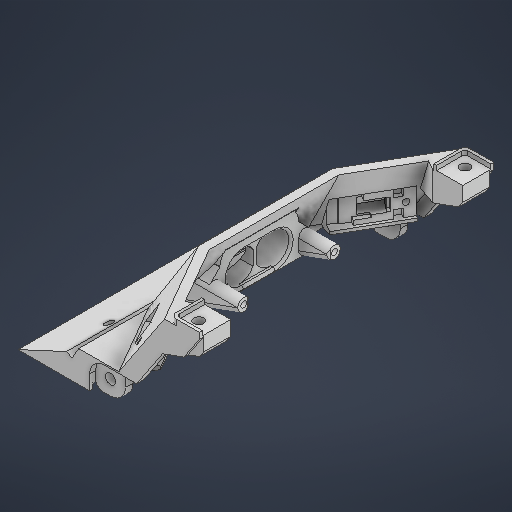
# Autodesk Inventor part: body-front
Saved by Autodesk Inventor 2025 (Build 290162000, 162)
## iProperties
Created: 2025-03-18
Part Number: body-front
Material: Všeobecné
Document SubType Name: Modeling
Designer: Simak
Density: 1 g/cm^3
Appearance: Výchozí
Author: Simak
Autodesk Inventor part; units mm, degrees
ref_plane "XZ Plane" through (0, 0, 0) normal (0, 1, 0) x (-1, 0, 0)
sketch "Náčrt1" plane through (0, 0, 0) normal (0, 0, 1) x (1, 0, 0)
  line L0 (29.0793, 0) -> (0, 0)
  line L1 (18.1093, 6.5703) -> (33.6572, 33.5)
  line L2 (33.6572, 33.5) -> (60.9683, 33.5)
  line L3 (60.9683, 33.5) -> (60.9683, 26.6) construction
  circle A0 centre (74.2183, 13.5) radius 16.5 construction
  line L4 (15.7407, 11.2018) -> (-8.2817, 0) construction
  line L5 (-8.2817, 0) -> (0, 0) construction
  line L6 (52.2183, 35.6) -> (89.7183, 35.6) construction
  line L7 (89.7183, 35.6) -> (89.7183, 34) construction
  line L8 (89.7183, 34) -> (52.2183, 34) construction
  line L9 (52.2183, 34) -> (52.2183, 35.6) construction
  line L10 (55.9683, 35.6) -> (55.9683, 34) construction
  circle A1 centre (74.2183, 15.5) radius 16.5
  circle A2 centre (74.2183, 11.5) radius 16.5
  line L11 (57.7183, 15.5) -> (57.7183, 11.5)
  line L12 (74.2183, 15.5) -> (74.2183, 13.5) construction
  line L13 (74.2183, 13.5) -> (74.2183, 11.5) construction
  line L14 (70.6632, 32.5) -> (65.9683, 29.7894)
  line L15 (70.6632, 33.5) -> (60.9683, 33.5)
  line L16 (70.6632, 33.5) -> (70.6632, 32.5)
  line L17 (62.0101, 26.6) -> (32.5602, 26.6)
  line L18 (10.0793, 4.2) -> (10.0793, 2.6) construction
  line L19 (20.5793, 4.2) -> (10.0793, 4.2) construction
  line L20 (11.4205, 8.6356) -> (13.8505, 3.4243) construction
  line L21 (13.8505, 3.4243) -> (12.7622, 0.4342) construction
  line L22 (12.7622, 0.4342) -> (19.5595, 3.6039) construction
  line L23 (19.5595, 3.6039) -> (16.5694, 4.6922) construction
  line L24 (16.5694, 4.6922) -> (14.1394, 9.9034) construction
  line L25 (14.1394, 9.9034) -> (11.4205, 8.6356) construction
  line L26 (10.0793, 2.6) -> (20.5793, 2.6) construction
  line L27 (20.5793, 2.6) -> (20.5793, 4.2) construction
  line L28 (20.5793, 4.2) -> (23.5793, 4.2) construction
  line L29 (23.5793, 4.2) -> (23.5793, 2.6) construction
  line L30 (23.5793, 2.6) -> (20.5793, 2.6) construction
  line L31 (19.5595, 3.6039) -> (21.24, 0) construction
  line L32 (0, 0) -> (16.3135, 7.6071)
  line L33 (16.3135, 7.6071) -> (18.1093, 6.5703)
  circle A3 centre (29.0793, 5) radius 5
  line L34 (22.9762, 10) -> (32.5602, 26.6)
  line L35 (22.9762, 10) -> (29.0793, 10)
  line L36 (15.7407, 11.2018) -> (17.2198, 8.0297) construction
  line L37 (17.2198, 8.0297) -> (16.3135, 7.6071) construction
  line L38 (22.9762, 10) -> (17.2027, 0)
  line L39 (34.0793, 5) -> (34.0793, 10.5)
  line L40 (34.0793, 10.5) -> (23.2649, 10.5)
  line L41 (32.5602, 26.6) -> (36.5439, 33.5)
  point P0 (90.7183, 13.5)
  dimension "d2" = 33
  dimension "d3" = 13.5
  dimension "d6" = 99
  dimension "d8" = 1.6
  dimension "d9" = 37.5
  dimension "d10" = 3.75
  dimension "d11" = 4
  dimension "d12" = 1
  dimension "d13" = 0.5
  dimension "d14" = 5
  dimension "d17" = 4
  dimension "d18" = 60
  dimension "d19" = 1
  dimension "d20" = 9
  dimension "d21" = 60
  dimension "d23" = 4.2
  dimension "d24" = 1.6
  dimension "d27" = 45
  dimension "d29" = 3
  dimension "d31" = 8
  dimension "d32" = 7.5
  dimension "d37" = 0.5
  dimension "d38" = 3
  dimension "d40" = 25
  dimension "d41" = 1
  dimension "d44" = 10.5
  dimension "d45" = 3.5
  dimension "d46" = 0.5
  dimension "d47" = 10
  dimension "d48" = 11.2018
  dimension "d49" = 0.5
  dimension "d50" = 2.5
  dimension "d58" = 19
  dimension "d59" = 1.5
  dimension "d65" = 2
  dimension "d80" = 18.361
  dimension "d86" = 10.5
  dimension "d336" = 45.139
  constraints: 85 end point, 15 perpendicular, 8 horizontal, 8 point on line, 6 point on circle, 5 tangent, 4 collinear, 4 parallel, 4 vertical, 3 equal length, 3 horizontal alignment, 2 centre point, 2 vertical alignment, 6 other
  measures "d3" distance from line of L0 L12.end
  measures "d6" horizontal distance of L4.end point (90.718, 13.5)
  measures "d8" distance of L6.end L7.end
  measures "d9" distance of L6.start L6.end
  measures "d10" distance between parallel lines of L9 L10
  measures "d12" distance from line of point (90.718, 13.5) L7
  measures "d13" distance between parallel lines of L8 L2
  measures "d14" distance between parallel lines of L10 L3
  measures "d17" distance of L13.end L12.start
  measures "d18" angle of L3 L14
  measures "d19" distance of L15.start L14.start
  measures "d20" distance between parallel lines of L6 L17
  measures "d21" angle of L0 L1
  measures "d23" distance between parallel lines of L0 L19
  measures "d24" distance of L18.start L18.end
  measures "d27" angle of L22 L23
  measures "d29" distance of L24.end L20.start
  measures "d31" distance from line of L24.end L22
  measures "d32" distance of L21.end L22.end
  measures "d37" distance from line of L31 L26.end
  measures "d38" distance of L19.start L28.end
  measures "d40" angle of L0 L32
  measures "d41" distance from line of L24 L32.end
  measures "d44" distance of L19.start L18.start
  measures "d45" distance between parallel lines of L32 L4
  measures "d46" distance between parallel lines of L4 L25
  measures "d47" diameter of A3
  measures "d48" distance from line of L0 L4.start
  measures "d49" distance edge to line of A3 L29
  measures "d50" distance between parallel lines of L1 L34
  measures "d58" distance from line of L0.end L36
  measures "d59" distance from line of L36.end L1
  measures "d65" distance between parallel lines of L36 L24
  measures "d80" horizontal distance of L4.end L18.end
  measures "d86" distance between parallel lines of L0 L40
  measures "d336" horizontal distance of A3.centre L12.end
extrude "Vysunutí1" add sketch "Náčrt1" along normal blind 49.5 contours L0 L38 L35 A3 | A3 | L0 L32 L33 L1 L2 L41 L34 L38 | L35 L34 L40 L39 A3
extrude "Vysunutí5" cut sketch "Náčrt1" along normal blind 44.9 contours L0 L38 L35 A3 | A3 | L35 L34 L40 L39 A3
ref_plane "Pracovní rovina1" through (0, 0, 0) normal (0.5, 0, 0.8660254) x (0, 1, 0)
sketch "Náčrt2" plane through (0, 0, 0) normal (0.5, 0, 0.8660254) x (0, 1, 0)
  line L0 (33.5, -20.7436) -> (10.5, -7.4646)
  line L1 (0, 0) -> (0, -14.898) projected
  line L2 (0, -2.7334) -> (0, -0.4334) projected
  line L3 (0, 24.75) -> (0, -0.4334) projected
  line L4 (0, 0) -> (0, 24.75) projected
  line L5 (33.5, -29.148) -> (33.5, -4.398) projected
  line L6 (0, 24.75) -> (0, 31.9222) construction
  line L7 (0, 0) -> (0, 7.1722) construction
  line L8 (33.5, -4.398) -> (6.5703, 9.0669) projected
  line L9 (10.5, -7.4646) -> (10.5, 7.102)
  line L10 (10.5, -4.5778) -> (33.5, -17.8569)
  line L11 (0, -14.898) -> (0, 7.552) projected
  line L12 (0, 7.552) -> (0, -2.7334) projected
  line L13 (14.8301, -7.0778) -> (10.5, 0.4222)
  circle A0 centre (10.5, 0.4222) radius 1.5 construction
  circle A1 centre (14.8301, -7.0778) radius 1.5 construction
  line L14 (10.5, -1.0778) -> (11.25, -0.8769) construction
  line L15 (14.0801, -5.7788) -> (13.5311, -6.3278) construction
  point P0 (11.2018, -13.6318)
  dimension "d69" = 60
  dimension "d74" = 2.5
  dimension "d79" = 36.5
  dimension "d83" = 10.5
  dimension "d90" = 3
  dimension "d92" = 5
  constraints: 16 end point, 12 point on line, 4 coincident, 4 point on circle, 2 centre point, 2 equal length, 2 vertical, 1 equal radius, 1 parallel
  measures "d69" angle of L2 L0
  measures "d74" distance between parallel lines of L0 L10
  measures "d79" vertical distance of L6.end L10.start
  measures "d83" distance between parallel lines of L9 L1
  measures "d90" diameter of A0
  measures "d92" distance of L10.start L13.end
extrude "Vysunutí2" add sketch "Náčrt2" along normal up to surface contours L0 L9 L10 L5 | L9 L13 L10 surface through (28.5277, 7.75, 49.5) normal (0, 0, 1)
extrude "Vysunutí3" cut sketch "Náčrt2" along normal through all contours L10 L13 L9 L8 L5 | L9 L13 L10
extrude "Vysunutí4" cut sketch "Náčrt2" along normal up to surface contours L0 L9 L10 L5 | L9 L13 L10 surface through (33.6572, 33.5, 0) normal (-0.8660254, 0.5, 0)
sketch "Náčrt4" plane through (0, 0, 49.5) normal (0, 0, 1) x (1, 0, 0)
  line L0 (36.8649, 10) -> (22.9762, 10)
  line L1 (0, 0) -> (29.0793, 0) projected
  line L2 (37.1982, 10.5) -> (34.0793, 10.5) projected
  line L3 (37.1982, 10.5) -> (36.8649, 10)
  line L4 (52.5315, 33.5) -> (37.1982, 10.5) projected
  line L5 (23.2649, 10.5) -> (17.2027, 0) construction
  line L6 (36.5439, 33.5) -> (17.2027, 0) projected
  line L7 (36.5439, 33.5) -> (23.2649, 10.5) construction
  line L8 (33.8649, 10.5) -> (20.3781, 10.5) projected
  line L9 (34.0793, 5) -> (34.0793, 10.5) construction
  line L10 (34.0793, 10.5) -> (31.2091, 10.5) projected
  line L11 (34.0793, 10.5) -> (28.0914, 10.5)
  point P0 (47.9382, 26.61)
  point P1 (23.5535, 10.5)
  point P2 (23.2649, 10.5)
  point P3 (23.2649, 10.5)
  dimension "d87" = 10
  constraints: 6 end point, 2 collinear, 1 horizontal, 1 parallel, 1 point on line
  measures "d87" distance between parallel lines of L1 L0
extrude "Vysunutí7" add sketch "Náčrt4" against normal up to surface surface through (6.4645, 10.5, -3.7323) normal (0.75, -0.5, -0.4330127)
sketch "Náčrt5" plane through (0, 0, 49.5) normal (0, 0, 1) x (1, 0, 0)
  line L0 (52.5315, 33.5) -> (36.8649, 10) projected
  line L1 (36.8649, 10) -> (39.8649, 10)
  line L2 (39.8649, 10) -> (55.5315, 33.5)
  line L3 (55.5315, 33.5) -> (52.5315, 33.5)
  line L4 (33.8649, 10.5) -> (20.3781, 10.5) projected
  line L5 (20.3781, 10.5) -> (18.1093, 6.5703) projected
  line L6 (18.1093, 6.5703) -> (16.3135, 7.6071) projected
  line L7 (16.3135, 7.6071) -> (0, 0) projected
  line L8 (0, 0) -> (29.0793, 0) projected
  arc A0 (29.0793, 0) -> (34.0793, 5) centre (29.0793, 5) ccw projected
  line L9 (34.0793, 5) -> (34.0793, 10) projected
  line L10 (34.0793, 10) -> (36.8649, 10) projected
  line L11 (52.5315, 33.5) -> (36.8649, 10) projected
  line L12 (49.1982, 33.5) -> (52.5315, 33.5) projected
  line L13 (49.1982, 33.5) -> (33.8649, 10.5) projected
  line L14 (34.0793, 10) -> (36.8649, 10) projected
  line L15 (34.0793, 10) -> (33.5315, 10)
  line L16 (22.9762, 10) -> (36.8649, 10) projected
  line L17 (33.8649, 10.5) -> (33.5315, 10)
  point P0 (36.8649, 10)
  dimension "d93" = 3
  constraints: 10 end point, 2 parallel, 1 collinear, 1 horizontal, 1 point on line
  measures "d93" distance of L2.end L0.start
extrude "Vysunutí8" add sketch "Náčrt5" against normal blind 2.5 contours L3 L2 L1 L0 | L0 L10 L15 L17 L13 L12
ref_plane "Pracovní rovina2" through (2.1131, -4.5315, 49.5) normal (-0.4226183, 0.9063078, 0) x (0.9063078, 0.4226183, 0)
sketch "Náčrt6" plane through (2.1131, -4.5315, 49.5) normal (-0.4226183, 0.9063078, 0) x (0.9063078, 0.4226183, 0)
  line L0 (15.5909, 4.6) -> (26.3548, 4.6) projected
  line L1 (25.0497, 24.0559) -> (25.0497, 4.6) projected
  line L2 (25.0497, 4.6) -> (15.5909, 4.6) projected
  line L3 (15.5909, 49.5) -> (15.5909, 4.6) projected
  line L4 (47.2777, 49.5) -> (15.5909, 49.5) projected
  line L5 (47.2777, 49.5) -> (47.2777, 27.6914) projected
  line L6 (47.2777, 27.6914) -> (25.0497, 24.0559) projected
  line L7 (0, 49.5) -> (15.5909, 49.5) projected
  line L8 (25.0497, 24.0559) -> (25.0497, 49.5)
  line L9 (15.5909, 4.6) -> (0, 4.6)
  line L10 (0, 49.5) -> (0, 0) projected
  constraints: 4 end point, 2 point on line, 1 horizontal, 1 perpendicular
extrude "Vysunutí9" cut sketch "Náčrt6" against normal through all contours L3 L4 L8 L1 L0 | L9 L10 L7 L3
sketch "Náčrt7" plane through (2.1131, -4.5315, 49.5) normal (0.4226183, -0.9063078, 0) x (0.9063078, 0.4226183, 0)
  line L0 (18, -49.5) -> (0, -49.5) projected
  line L1 (0, -49.5) -> (0, 0) projected
  point P0 (15.5, -49.5)
  point P1 (15.5, -16.5)
  dimension "d99" = 33
  dimension "d100" = 15.5
  constraints: 1 point on line, 1 vertical alignment
  measures "d99" distance from line of L0 point (15.5, -16.5)
  measures "d100" distance from line of point (15.5, -49.5) L1
hole "Díra1" at (16.1609, 2.019, 0) at (16.1609, 2.019, 33) direction (-0.4226183, 0.9063078, 0) diameter 3 end through all countersink diameter 7 countersink angle 90
sketch "Náčrt9" plane through (0, 0, 49.5) normal (0, -1, 0) x (1, 0, 0)
  line L0 (23.5793, -1) -> (10.0793, -1)
  line L1 (10.0793, -1) -> (10.0793, -8)
  line L2 (10.0793, -8) -> (20.5793, -8)
  line L3 (20.5793, -8) -> (20.5793, -25)
  line L4 (20.5793, -25) -> (17.5793, -28)
  line L5 (17.5793, -28) -> (17.5793, -38)
  line L6 (17.5793, -38) -> (20.5793, -41)
  line L7 (20.5793, -49.5) -> (20.5793, -41)
  line L8 (10.0793, -2) -> (23.5793, -2)
  circle A0 centre (20.5793, -33) radius 1.5
  line L9 (20.5793, -33) -> (23.5793, -33) construction
  line L10 (20.5793, -33) -> (17.5793, -33) construction
  line L11 (26.5793, -55.5) -> (26.5793, -43.5)
  line L12 (23.5793, -40.5) -> (23.5793, -1)
  line L13 (33.6572, -49.5) -> (18.1093, -49.5) projected
  line L14 (23.5793, -40.5) -> (26.5793, -43.5)
  ellipse E0 centre (15.3156, -49.5) end of major axis (15.3156, -48) minor radius 1.3595 (16.6751, -49.5) -> (13.9562, -49.5) ccw projected
  ellipse E1 centre (15.3156, -16.5) end of major axis (15.3156, -15) minor radius 1.3595 projected
  line L15 (15.3156, -16.5) -> (20.5793, -33) construction
  line L16 (15.3156, -49.5) -> (20.5793, -33) construction
  line L17 (23.5793, -1) -> (24.0793, -1)
  line L18 (24.0793, -1) -> (24.0793, -4.6)
  line L19 (11.831, -4.6) -> (29.0793, -4.6) projected
  line L20 (11.5793, -2) -> (11.5793, -1)
  point P0 (0, -49.5)
  point P1 (26.5793, -49.5)
  point P2 (10.0793, -49.5)
  point P3 (10.0793, -49.5)
  point P4 (10.0793, -49.5)
  point P5 (23.5793, -4.6)
  dimension "d108" = 3
  dimension "d109" = 135
  dimension "d110" = 10
  dimension "d111" = 1
  dimension "d112" = 10.5
  dimension "d113" = 6
  dimension "d114" = 12
  dimension "d115" = 3
  dimension "d116" = 3
  dimension "d118" = 3
  dimension "d119" = 48.5
  dimension "d121" = 45
  dimension "d122" = 16.5
  dimension "d125" = 0.5
  dimension "d129" = 1.5
  constraints: 38 end point, 9 point on line, 6 perpendicular, 3 equal length, 2 midpoint, 2 parallel, 1 centre point, 1 collinear, 1 horizontal, 1 vertical, 1 vertical alignment, 2 other
  measures "d108" diameter of A0
  measures "d109" angle of L5 L4
  measures "d110" distance of L5.start L6.start
  measures "d111" distance between parallel lines of L8 L0
  measures "d112" distance of L2.start L2.end
  measures "d113" distance between parallel lines of L2 L8
  measures "d114" distance of L11.start L11.end
  measures "d115" distance between parallel lines of L7 L12
  measures "d116" distance between parallel lines of L7 L5
  measures "d118" distance between parallel lines of L12 L11
  measures "d119" distance from line of L7.start L0
  measures "d121" angle of L12 L14
  measures "d122" distance between parallel lines of L13 L9
  measures "d125" distance of L12.end L17.end
  measures "d129" distance between parallel lines of L1 L20
extrude "Vysunutí10" cut sketch "Náčrt9" against normal blind 4.2 contours L12 L8 L20 L0 | L17 L18 L19 L12 | L12 L14 L11 L13 L7 L6 L5 L4 L3 L2 L1 L8 | A0
sketch "Náčrt10" plane through (0, 4.2, 49.5) normal (0, -1, 0) x (1, 0, 0)
  line L0 (10.0793, -2) -> (11.5793, -2) projected
  line L1 (11.5793, -2) -> (11.5793, -1) projected
  line L2 (11.5793, -1) -> (10.0793, -1)
  line L3 (10.0793, -1) -> (10.0793, -2)
  point P0 (0, -49.5)
  constraints: 4 end point, 1 horizontal, 1 perpendicular
extrude "Vysunutí11" cut sketch "Náčrt10" along normal blind 2
sketch "Náčrt11" plane through (0, 4.2, 49.5) normal (0, -1, 0) x (1, 0, 0)
  line L0 (23.5793, -40.5) -> (23.5793, -1) projected
  line L1 (20.5793, -49.5) -> (20.5793, -41) projected
  line L2 (17.5793, -38) -> (20.5793, -41) projected
  line L3 (20.5793, -25) -> (17.5793, -28) projected
  line L4 (20.5793, -8) -> (20.5793, -25) projected
  line L5 (10.0793, -8) -> (20.5793, -8) projected
  line L6 (23.5793, -40.5) -> (26.5793, -43.5) projected
  line L7 (26.5793, -55.5) -> (26.5793, -43.5) projected
  circle A0 centre (20.5793, -33) radius 1.5 projected
  circle A1 centre (20.5793, -33) radius 3
  line L8 (19.6275, -25.9518) -> (19.6275, -40.0482) projected
  line L9 (20.5793, -30) -> (19.6275, -30)
  line L10 (20.5793, -36) -> (19.6275, -36)
  point P0 (0, -49.5)
  point P1 (19.6275, -34.1594)
  point P2 (19.6275, -31.8406)
  point P3 (19.6275, -35.845)
  point P4 (19.6275, -30.155)
  constraints: 4 end point, 3 tangent, 2 perpendicular, 2 point on circle, 2 point on line, 1 centre point, 1 coincident
extrude "Vysunutí12" add sketch "Náčrt11" against normal up to next contours A0 L8 A1 | L8 L9 A1 | A1 L10 L8 picked at (23.0542, -33.2225)
extrude "Vysunutí13" cut sketch "Náčrt11" against normal through all contours A0 L8 | L8 A0
sketch "Náčrt12" plane through (0, 0, 0) normal (0, 0, -1) x (-1, 0, 0)
  line L0 (-43.5793, 29.075) -> (-43.5793, 7.825)
  line L1 (-43.5793, 7.825) -> (-32.8059, 8.0131)
  arc A0 (-32.8059, 8.0131) -> (-31.5793, 9.2612) centre (-32.8277, 9.2612) ccw
  line L2 (-31.5793, 9.2612) -> (-31.5793, 12)
  line L3 (-31.5793, 12) -> (-30.0793, 12)
  line L4 (-30.0793, 12) -> (-30.0793, 22.65)
  line L5 (-30.0793, 22.65) -> (-31.5793, 22.65)
  line L6 (-31.5793, 22.65) -> (-31.5793, 25.3888)
  arc A1 (-31.5793, 25.3888) -> (-32.8059, 26.6369) centre (-32.8277, 25.3888) ccw
  line L7 (-32.8059, 26.6369) -> (-43.5793, 26.825)
  line L8 (-35.0793, 26.6766) -> (-35.0793, 29.075)
  line L9 (-35.0793, 29.075) -> (-43.5793, 29.075)
  line L10 (-41.5793, 17.825) -> (-41.5793, 15.825)
  arc A2 (-34.0793, 5) -> (-29.0793, 0) centre (-29.0793, 5) ccw projected
  line L11 (-18.1093, 6.5703) -> (-16.3135, 7.6071) construction
  line L12 (-17.2198, 8.0297) -> (-16.3135, 7.6071) construction
  line L13 (-17.2198, 8.0297) -> (-15.7407, 11.2018) construction
  line L14 (-15.7407, 11.2018) -> (8.2817, 0) construction
  line L15 (8.2817, 0) -> (0, 0) construction
  line L16 (-12.6883, 5.9167) -> (0, 0) construction
  point P0 (-41.5793, 16.825)
  point P1 (-30.0793, 17.325)
  dimension "d137" = 10.65
  dimension "d138" = 0.5
  dimension "d139" = 2
  dimension "d140" = 11.5
  dimension "d141" = 1.5
  dimension "d145" = 2
  dimension "d146" = 91
  dimension "d147" = 11.75
  dimension "d148" = 13.5
  dimension "d149" = 8.5
  dimension "d150" = 1.75
  dimension "d152" = 9
  dimension "d153" = 10
  dimension "d154" = 19
  dimension "d155" = 3.5
  dimension "d156" = 12
  dimension "d157" = 1
  constraints: 30 end point, 7 perpendicular, 4 point on circle, 4 point on line, 4 tangent, 2 centre point, 2 midpoint, 2 vertical, 1 equal radius, 1 horizontal, 1 parallel
  measures "d137" distance of L3.end L4.end
  measures "d138" vertical distance of point (-41.579, 16.825) point (-30.079, 17.325)
  measures "d139" distance of L10.start L10.end
  measures "d140" distance between parallel lines of L10 L4
  measures "d141" distance of L2.end L3.end
  measures "d145" angle of L1 L7
  measures "d146" angle of L4 L7
  measures "d147" distance from line of point (-30.079, 17.325) L9
  measures "d148" distance between parallel lines of L4 L0
  measures "d149" distance of L8.end L0.start
  measures "d150" distance of L6.end L7.start
  measures "d152" vertical distance of point (-41.579, 16.825) L0.end
  measures "d153" vertical distance of L7.end point (-41.579, 16.825)
  measures "d154" distance of L15.end L12.start
  measures "d155" distance of L12.start L13.end
  measures "d156" distance from line of L15.end L3
  measures "d157" distance from line of L4 A2.centre
ref_plane "Pracovní rovina3" through (41.5793, 16.825, 0) normal (1, 0, 0) x (0, 1, 0)
ref_plane "Pracovní rovina4" through (31.5793, 22.65, 0) normal (-1, 0, 0) x (0, -1, 0)
sketch "Náčrt13" plane through (41.5793, 16.825, 0) normal (1, 0, 0) x (0, 1, 0)
  line L0 (1, 0) -> (-1, 0) projected
  circle A0 centre (0, 15.25) radius 1
  circle A1 centre (0, 15.25) radius 2
  line L1 (0, 17.25) -> (0, 13.25) construction
  line L2 (0, 17.25) -> (-3, 17.25)
  circle A2 centre (-3, 15.25) radius 2
  line L3 (-3, 13.25) -> (0, 13.25)
  point P0 (-16.825, 0)
  point P1 (0, 0)
  dimension "d158" = 2
  dimension "d159" = 15.25
  dimension "d160" = 4
  dimension "d173" = 3
  constraints: 6 end point, 4 point on circle, 3 centre point, 3 tangent, 2 coincident, 2 horizontal, 2 midpoint, 1 equal radius, 1 horizontal alignment, 1 vertical, 1 vertical alignment
  measures "d158" diameter of A0
  measures "d159" distance from line of L0 A0.centre
  measures "d160" diameter of A1
  measures "d173" distance of A0.centre A2.centre
ref_plane "Pracovní rovina6" through (41.5793, 16.825, 17.25) normal (0.9396926, 0.3420201, 0) x (0, 0, -1)
sketch "Náčrt15" plane through (41.5793, 16.825, 17.25) normal (0.9396926, 0.3420201, 0) x (0, 0, -1)
  circle A0 centre (2, 0) radius 2
  line L0 (2, -2) -> (4, -2)
  line L1 (4, -2) -> (4, 0)
  point P0 (17.25, -1.5894)
  dimension "d166" = 4
  constraints: 4 end point, 2 point on circle, 2 tangent, 1 centre point, 1 coincident, 1 horizontal, 1 perpendicular
  measures "d166" diameter of A0
extrude "Vysunutí14" add sketch "Náčrt15" against normal up to next
extrude "Vysunutí19" cut sketch "Náčrt15" against normal up to surface contours L1 L0 A0 surface through (31.5793, 22.65, 0) normal (-1, 0, 0)
extrude "Vysunutí15" add sketch "Náčrt13" against normal up to next contours A2 A1 | A2 A1 picked at (-0.9946, 14.1304) picked at (-1.6474, 15.0909)
ref_plane "Pracovní rovina7" through (41.5793, 16.825, 13.25) normal (0, 0, -1) x (-1, 0, 0)
sketch "Náčrt16" plane through (41.5793, 16.825, 13.25) normal (0, 0, -1) x (-1, 0, 0)
  line L0 (15.8174, -2) -> (13.508, 2) projected
  line L1 (0, 0) -> (0, 0) projected
  line L2 (0, 0) -> (0, 0) projected
  line L3 (0, 0) -> (0, 0) projected
  line L4 (0, 0) -> (0, 0) projected
  line L5 (18.0706, -5.9026) -> (18.5637, -6.7566) projected
  line L6 (5.0354, 16.675) -> (22.3377, -13.2935) projected
  line L7 (0, 2) -> (13.508, 2) projected
  line L8 (-0.684, -1.8794) -> (18.2728, -8.7791) projected
  line L9 (0, 2) -> (0, 0) projected
  line L10 (0, 0) -> (-0.684, -1.8794) projected
  line L11 (0, 0) -> (18.5637, -6.7566)
  line L12 (0, 0) -> (0, 1) projected
  line L13 (0, 0) -> (14.6627, 0)
  line L14 (10, -3.6397) -> (18.5637, -6.7566) projected
  line L15 (10, -5.7681) -> (18.2728, -8.7791) projected
  line L16 (10, -3.6397) -> (10, -5.7681) projected
  point P0 (41.5793, -16.825)
  point P1 (17.8681, -8.15)
  point P2 (22.3377, -13.2935)
  point P3 (14.6627, 0)
  constraints: 4 end point, 2 parallel, 4 other
extrude "Vysunutí16" add sketch "Náčrt16" against normal blind 4 contours L6 L5 L11 L13 L0
extrude "Vysunutí17" cut sketch "Náčrt13" along normal through all contours A0 | A2 A1 | A2 A1 | A2 L2 A1 | A1 A2 | A1 L3 A2
extrude "Vysunutí18" cut sketch "Náčrt13" against normal through all contours A0
sketch "Náčrt17" plane through (31.5793, 22.65, 0) normal (-1, 0, 0) x (0, -1, 0)
  circle A0 centre (5.325, 5.325) radius 5.325
  circle A1 centre (5.825, 15.25) radius 1 projected
  line L0 (-10.85, 0) -> (19.1185, 0) projected
  line L1 (14.825, 13.25) -> (-4.175, 13.25)
  line L2 (-4.175, 13.25) -> (-4.175, -13.25)
  line L3 (-4.175, -13.25) -> (14.825, -13.25)
  line L4 (14.825, -13.25) -> (14.825, 13.25)
  arc A2 (5.825, 17.25) -> (5.825, 13.25) centre (5.825, 15.25) ccw projected
  arc A3 (0.825, 13.25) -> (-4.175, 8.25) centre (0.825, 8.25) ccw
  arc A4 (14.825, 10.25) -> (11.825, 13.25) centre (11.825, 10.25) ccw
  line L5 (3.825, 15.25) -> (3.825, 13.25)
  arc A5 (5.825, 17.25) -> (5.825, 13.25) centre (5.825, 15.25) ccw projected
  line L6 (10.65, 5.325) -> (10.65, 0)
  line L7 (0, 5.325) -> (0, 0)
  line L8 (7.7806, 0.6) -> (2.8694, 0.6)
  line L9 (-2.7105, 11.7855) -> (-6.175, 8.3211)
  line L10 (-6.175, 8.3211) -> (-6.175, 0)
  line L11 (4.4108, 16.6642) -> (0.9966, 13.25)
  point P0 (22.65, 0)
  point P1 (-5.825, 13.25)
  point P2 (5.325, -13.25)
  point P3 (-4.175, 0)
  point P4 (5.325, 0)
  point P5 (14.825, 0)
  point P6 (-5.825, 13.25)
  point P7 (-4.175, 10.3211)
  point P8 (4.4108, 16.6642)
  dimension "d178" = 0.5
  dimension "d179" = 10.65
  dimension "d180" = 19
  dimension "d181" = 26.5
  dimension "d182" = 10
  dimension "d183" = 6
  dimension "d191" = 0.6
  dimension "d199" = 2
  dimension "d262" = 45
  constraints: 22 end point, 11 point on circle, 11 tangent, 9 point on line, 4 perpendicular, 3 centre point, 3 parallel, 2 horizontal, 1 midpoint, 1 vertical alignment
  measures "d178" horizontal distance of A1.centre A0.centre
  measures "d179" diameter of A0
  measures "d180" distance of L1.start L1.end
  measures "d181" distance of L3.end L1.start
  measures "d182" diameter of A3
  measures "d183" diameter of A4
  measures "d191" distance between parallel lines of L0 L8
  measures "d199" distance between parallel lines of L2 L10
  measures "d262" angle of L1 L11
extrude "Vysunutí20" add sketch "Náčrt17" along normal up to next contours A0 L7 L0 L2 A3 L1 A4 L4 L6 | L0 L10 L9 L2 | L1 L5 A2 | L1 L11 A2 L5
extrude "Vysunutí22" cut sketch "Náčrt17" along normal through all contours A0 L8 | L6 L0 A0 | A0 L0 L7 | A0 L8
ref_plane "Pracovní rovina8" through (20.2744, 5.3203, 0) normal (-0.8660254, 0.5, 0) x (0, 0, 1)
extrude "Vysunutí26" add sketch "Náčrt17" along normal up to surface contours L6 L0 A0 | A0 L0 L7 | A0 L8 surface through (20.2744, 5.3203, 0) normal (-0.8660254, 0.5, 0) picked at (4.7674, 0.4898)
ref_plane "Pracovní rovina9" through (27.3929, 22.65, 0) normal (1, 0, 0) x (0, 1, 0)
extrude "Vysunutí27" add sketch "Náčrt17" along normal up to surface (4.1864 mm away) contours L6 L0 A0 | A0 L0 L7 | A0 L8 picked at (4.7674, 0.4898)
extrude "Vysunutí37" cut sketch "Náčrt17" along normal blind 1.5 contours L6 L0 A0 | A0 L0 L7 | A0 L8 picked at (4.7674, 0.4898)
sketch "Náčrt18" plane through (31.5793, 21.825, 13.25) normal (0, 0, -1) x (-1, 0, 0)
  line L0 (0, -8.6397) -> (0, -5) projected
  line L1 (0.6373, -11) -> (10.1194, -14.4512) projected
  line L2 (8.1268, -11) -> (10.1194, -14.4512) projected
  line L3 (-10, -5) -> (0, -5) projected
  line L4 (0, -8.6397) -> (-10, -5) projected
  line L5 (0.6373, -11) -> (8.1268, -11) projected
  line L6 (0, -14) -> (9.8589, -14) projected
  point P0 (31.5793, -21.825)
  point P1 (8.8797, -14)
extrude "Vysunutí21" add sketch "Náčrt18" along normal up to surface (13.25 mm away) contours L5 L2 L6 L1 | L6 L2 L1
sketch "Náčrt20" plane through (0, 0, 0) normal (0, 0, -1) x (-1, 0, 0)
  line L0 (-32.8205, 27.0509) -> (-31.5793, 26.5991)
  line L1 (-41.5793, 14.6966) -> (-23.3065, 8.0459) projected
  line L2 (-31.5793, 24.9011) -> (-31.5793, 12) projected
  line L3 (-36.5439, 33.5) -> (-19.2416, 3.5315) projected
  line L4 (-31.5793, 11.0569) -> (-30.9421, 10.825) projected
  line L5 (-30.9421, 10.825) -> (-22.6996, 7.825) projected
  line L6 (-31.5793, 7.825) -> (-22.6996, 7.825) projected
  line L7 (-31.5793, 12) -> (-31.5793, 7.825) projected
  point P0 (0, 0)
  point P1 (-31.5793, 26.825)
  point P2 (-31.5793, 26.825)
  point P3 (-31.5793, 26.825)
  point P4 (-32.1999, 26.825)
  point P5 (-21.4599, 7.3738)
  point P6 (-21.7204, 7.825)
  constraints: 2 end point, 1 horizontal alignment, 1 midpoint, 1 parallel, 1 point on line
extrude "Vysunutí25" cut sketch "Náčrt20" against normal up to next
ref_plane "Pracovní rovina10" through (43.816, 33.5, 34.4043) normal (0.5, 0, 0.8660254) x (0, 1, 0)
sketch "Náčrt21" plane through (43.816, 33.5, 34.4043) normal (0.5, 0, 0.8660254) x (0, 1, 0)
  line L0 (-11.675, 7.2406) -> (-20.675, 7.2406)
  line L1 (-20.675, 7.2406) -> (-20.675, 6.2406)
  line L2 (-20.675, 6.2406) -> (-11.675, 6.2406)
  line L3 (-11.675, 6.2406) -> (-11.675, 7.2406)
  line L4 (0, 0) -> (-23.5, 13.5677) projected
  ellipse E0 centre (-16.175, -3.9423) end of major axis (-10.85, -3.9423) minor radius 2.6625 (-10.85, -3.9423) -> (-21.5, -3.9423) ccw projected
  point P0 (-33.5, 20.7436)
  point P1 (-16.175, -3.9423)
  point P2 (-16.175, 6.2406)
  point P3 (-11.675, 6.7406)
  dimension "d207" = 1
  dimension "d208" = 9
  dimension "d209" = 0.5
  constraints: 8 end point, 2 midpoint, 2 parallel, 1 horizontal, 1 perpendicular, 1 point on line, 1 vertical alignment, 1 other
  measures "d207" distance of L2.end L0.start
  measures "d208" distance of L1.end L2.end
  measures "d209" distance of L0.start point (-11.675, 6.741)
ref_plane "Pracovní rovina11" through (37.5455, 21.825, 38.0246) normal (-0.8660254, 0, 0.5) x (0, -1, 0)
sketch "Náčrt22" plane through (37.5455, 21.825, 38.0246) normal (-0.8660254, 0, 0.5) x (0, -1, 0)
  line L0 (9, 0) -> (0, 0) projected
  line L1 (0, 6.4511) -> (9, 6.4511)
  line L2 (9, 6.4511) -> (9, -15.1489)
  line L3 (9, -15.1489) -> (0, -15.1489)
  line L4 (0, -15.1489) -> (0, 6.4511)
  line L5 (-11.675, -14.5442) -> (11.825, -18.1797) projected
  line L6 (-11.675, 14.5442) -> (11.825, 6.7109) projected
  line L7 (9, 6.4511) -> (9, 7.6526) construction
  line L8 (0, -15.1489) -> (0, -16.3504) construction
  line L9 (3.3, -6.6489) -> (3.3, -1.8489)
  line L10 (3.3, -1.8489) -> (5.7, -1.8489)
  line L11 (5.7, -1.8489) -> (5.7, -6.6489)
  line L12 (5.7, -6.6489) -> (3.3, -6.6489)
  line L13 (5.7, -4.2489) -> (9, -4.2489) construction
  line L14 (3.3, -4.2489) -> (0, -4.2489) construction
  circle A0 centre (4.5, 3.9111) radius 1
  line L15 (2.3, -0.8489) -> (2.3, -7.6489)
  line L16 (2.3, -7.6489) -> (6.7, -7.6489)
  line L17 (6.7, -7.6489) -> (6.7, -0.8489)
  line L18 (6.7, -0.8489) -> (2.3, -0.8489)
  point P0 (21.825, -51.703)
  point P1 (4.5, -1.8489)
  dimension "d211" = 9
  dimension "d212" = 21.6
  dimension "d213" = 4.8
  dimension "d214" = 2.4
  dimension "d215" = 8.3
  dimension "d216" = 2
  dimension "d217" = 2.54
  dimension "d222" = 1
  constraints: 32 end point, 6 parallel, 6 point on line, 4 perpendicular, 3 midpoint, 3 vertical, 2 equal length, 1 centre point, 1 horizontal, 1 vertical alignment, 3 other
  measures "d211" distance of L2.end L3.end
  measures "d212" distance of L1.end L2.end
  measures "d213" distance of L10.end L11.end
  measures "d214" distance of L9.end L10.end
  measures "d215" distance between parallel lines of L1 L10
  measures "d216" diameter of A0
  measures "d217" distance from line of L1 A0.centre
  measures "d222" distance between parallel lines of L9 L15
extrude "Vysunutí28" cut sketch "Náčrt22" against normal up to next contours L2 L3 L4 L0 | L0 L4 L1 L2 | L9 L10 L11 L12 | A0 | L18 L17 L16 L15
extrude "Vysunutí29" add sketch "Náčrt22" along normal up to next contours L2 L3 L4 L0 | L0 L4 L1 L2
extrude "Vysunutí30" cut sketch "Náčrt22" along normal through all contours L9 L10 L11 L12 | A0 | L18 L17 L16 L15
ref_plane "Pracovní rovina12" through (35.4211, 15.125, 34.3449) normal (0.5, 0, 0.8660254) x (0.8660254, 0, -0.5)
ref_plane "Pracovní rovina13" through (33.7211, 17.325, 31.4005) normal (0, -1, 0) x (0.8660254, 0, -0.5)
sketch "Náčrt23" plane through (35.4211, 15.125, 34.3449) normal (0.5, 0, 0.8660254) x (0.8660254, 0, -0.5)
  line L0 (0, 4.4) -> (-3.7147, 4.4) projected
  line L1 (0, 0) -> (-6.255, 0) projected
  line L2 (0, 0) -> (-6.9639, -1.2279)
  line L3 (4.3538, 18.375) -> (-8.9252, -4.625) projected
  line L4 (0, 4.4) -> (-3.3714, 4.9945)
  point P0 (-13.5031, -15.125)
  dimension "d225" = 10
  dimension "d226" = 10
  constraints: 4 end point, 2 point on line
  measures "d225" angle of L0 L4
  measures "d226" angle of L1 L2
extrude "Vysunutí31" cut sketch "Náčrt23" along normal mid plane 6.8
sketch "Náčrt24" plane through (33.7211, 17.325, 31.4005) normal (0, -1, 0) x (0.8660254, 0, -0.5)
  line L0 (-6.9639, 6.8) -> (0, 6.8) projected
  line L1 (0, 0) -> (-6.9639, 0) projected
  line L2 (0, 6.8) -> (-6.9639, 8.0279)
  line L3 (-6.9639, 6.8) -> (-6.9639, 0) projected
  line L4 (-6.9639, 6.8) -> (-6.9639, 8.0279)
  line L5 (0, 6.8) -> (0, 0) projected
  line L6 (0, 0) -> (-6.9639, -1.2279)
  line L7 (-6.9639, 0) -> (-6.9639, -1.2279)
  point P0 (-13.5031, -44.0541)
  dimension "d229" = 10
  dimension "d230" = 10
  constraints: 8 end point, 2 vertical
  measures "d229" angle of L0 L2
  measures "d230" angle of L1 L6
extrude "Vysunutí32" cut sketch "Náčrt24" along normal up to surface surface through (29.3901, 13.8971, 37.8269) normal (0.1503837, -0.9848078, -0.0868241)
extrude "Vysunutí33" cut sketch "Náčrt24" against normal up to surface surface through (35.4211, 19.525, 34.3449) normal (0.1503837, 0.9848078, -0.0868241)
sketch "Náčrt25" plane through (37.5455, 21.825, 38.0246) normal (0.8660254, 0, -0.5) x (-0.5, 0, -0.8660254)
  line L0 (15.1489, -9) -> (15.1489, 0)
  line L1 (15.1489, 0) -> (-6.4511, 0)
  line L2 (-6.4511, 0) -> (-6.4511, -9)
  line L3 (15.1489, -9) -> (15.1489, -9)
  line L4 (15.1489, 0) -> (15.1489, -9)
  line L5 (4.6989, -6.5) -> (-0.9511, -6.5)
  line L6 (-6.4511, -9) -> (15.1489, -9)
  line L7 (-0.9511, -6.5) -> (-0.9511, -9)
  line L8 (4.6989, -6.5) -> (4.6989, -9)
  line L9 (-3.2011, -9) -> (-3.2011, 0)
  line L10 (-3.2011, -6.25) -> (-0.2011, -6.25)
  line L11 (-0.2011, -6.25) -> (-0.2011, -2.75)
  line L12 (-0.2011, -2.75) -> (-3.2011, -2.75)
  line L13 (-0.9511, -6.5) -> (-0.9511, -6.25)
  line L14 (-0.2011, -6.25) -> (-0.2011, -6.5)
  line L15 (-0.9511, -2.75) -> (-0.9511, 0)
  line L16 (-0.9511, -2.5) -> (6.5489, -2.5)
  line L17 (-6.4511, 0) -> (15.1489, 0)
  line L18 (6.5489, -2.5) -> (6.5489, 0)
  line L19 (12.3989, 0) -> (12.3989, -9)
  line L20 (-0.2011, -2.75) -> (-0.2011, -2.5)
  line L21 (4.6989, -7.5) -> (9.0489, -7.5)
  line L22 (9.0489, -7.5) -> (9.0489, -9)
  line L23 (0.8489, -2.3) -> (0.8489, -6.7) projected
  line L24 (7.6489, -2.3) -> (0.8489, -2.3) projected
  line L25 (7.6489, -6.7) -> (7.6489, -2.3) projected
  line L26 (0.8489, -6.7) -> (7.6489, -6.7) projected
  circle A0 centre (-3.9111, -4.5) radius 1 projected
  line L27 (15.1489, 0) -> (15.1489, -0.866) projected
  line L28 (-6.4511, 0) -> (15.1489, 0) projected
  line L29 (-6.4511, -0.866) -> (-6.4511, 0) projected
  line L30 (-6.4511, -9) -> (-6.4511, -0.866) projected
  line L31 (15.1489, -9) -> (-6.4511, -9) projected
  line L32 (15.1489, -0.866) -> (15.1489, -9) projected
  line L33 (15.1489, -9) -> (-6.4511, -9) projected
  line L34 (-6.4511, 0) -> (15.1489, 0) projected
  circle A1 centre (-3.9111, -4.5) radius 1 projected
  point P0 (51.703, -21.825)
  point P1 (4.6989, -6.7)
  point P2 (6.5489, 0)
  point P3 (6.5489, -2.3)
  point P4 (0.8489, -6.5)
  point P5 (0.8489, -2.5)
  dimension "d236" = 5.5
  dimension "d237" = 3.25
  dimension "d239" = 2.75
  dimension "d240" = 6.25
  dimension "d241" = 2.5
  dimension "d242" = 2.75
  dimension "d243" = 11.15
  dimension "d244" = 15.5
  dimension "d246" = 13
  dimension "d248" = 2.54
  dimension "d249" = 1.5
  dimension "d250" = 2.5
  dimension "d251" = 2.75
  constraints: 46 end point, 18 point on line, 8 perpendicular, 6 collinear, 6 parallel
  measures "d236" distance between parallel lines of L2 L7
  measures "d237" distance between parallel lines of L2 L9
  measures "d239" distance between parallel lines of L12 L1
  measures "d240" distance between parallel lines of L2 L11
  measures "d241" distance between parallel lines of L1 L16
  measures "d242" distance between parallel lines of L3 L19
  measures "d243" distance between parallel lines of L2 L8
  measures "d244" distance between parallel lines of L2 L22
  measures "d246" distance between parallel lines of L2 L18
  measures "d248" distance from line of L2 A0.centre
  measures "d249" distance of L22.start L22.end
  measures "d250" distance of L5.start L8.end
  measures "d251" distance between parallel lines of L6 L10
extrude "Vysunutí34" cut sketch "Náčrt25" against normal blind 1.5 contours L6 L22 L21 L8 L26 L25 L24 L18 L1 L19 | L6 L9 L10 L13 L7 | L15 L12 L9 L1 | L14 L11 L20 L16 L23 L5
extrude "Vysunutí35" cut sketch "Náčrt25" against normal blind 2 contours L6 L19 L1 L0
sketch "Náčrt26" plane through (40.7711, 12.825, 43.6114) normal (0.5, 0, 0.8660254) x (0.8660254, 0, -0.5)
  line L0 (0, 0) -> (0, 2.75) projected
  line L1 (0, 0) -> (1, 0)
  line L2 (1, 0) -> (1, -1)
  line L3 (7.2406, 20.675) -> (-6.3272, -2.825) projected
  line L4 (-2, 0) -> (-4.6962, 0) projected
  line L5 (-2, 0) -> (-1.5, 0) projected
  line L6 (-1.5, 0) -> (0, 0) projected
  line L7 (0, 0) -> (-1.5, 0) projected
  line L8 (-1.5, 0) -> (0, 0) projected
  line L9 (0, 0) -> (-4.6962, 0) projected
  line L10 (-2, 0) -> (-4.6962, 0) projected
  line L11 (1, -1) -> (-4.0141, -2.825)
  line L12 (-4.0141, -2.825) -> (-6.3272, -2.825)
  point P0 (-13.5031, -12.825)
  point P1 (-2, 0)
  dimension "d256" = 1
  dimension "d257" = 1
  dimension "d274" = 70
  constraints: 8 end point, 2 horizontal, 1 perpendicular
  measures "d256" distance of L0.start L1.end
  measures "d257" distance of L1.end L2.end
  measures "d274" angle of L2 L11
extrude "Vysunutí36" add sketch "Náčrt26" against normal up to surface (21.6 mm away)
fillet "Zaoblení1" radius 0.75 3 edges at (31.5793, 12, 2.6625) (31.5793, 22.65, 2.6625) (31.5793, 17.325, 10.65)
sketch "Náčrt27" plane through (0, 0, 0) normal (0, 0, -1) x (-1, 0, 0)
  circle A0 centre (-32.8168, 25.5876) radius 1.2374
  line L0 (-31.5793, 24.9011) -> (-31.5793, 23.4) projected
  line L1 (-30.8293, 12) -> (-30.8293, 22.65) projected
  line L2 (-30.0793, 12) -> (-30.8293, 12) projected
  line L3 (-30.0793, 12) -> (-30.0793, 14.8694) projected
  line L4 (-30.0793, 14.8694) -> (-25.7875, 14.8694) projected
  line L5 (-25.7875, 14.8694) -> (-24.1309, 12) projected
  line L6 (-24.1309, 12) -> (-21.2441, 12) projected
  line L7 (-27.3929, 22.65) -> (-21.2441, 12) projected
  line L8 (-27.3929, 19.7806) -> (-27.3929, 22.65) projected
  line L9 (-30.0793, 19.7806) -> (-27.3929, 19.7806) projected
  line L10 (-30.0793, 19.7806) -> (-30.0793, 22.65) projected
  line L11 (-30.0793, 22.65) -> (-30.8293, 22.65) projected
  line L12 (-31.5793, 24.9011) -> (-31.5793, 25.5876)
  line L13 (-36.5439, 33.5) -> (-31.5793, 24.9011) projected
  point P0 (0, 0)
  point P1 (-30.8293, 17.325)
  point P2 (-32.8168, 26.825)
  point P3 (-31.6858, 25.0854)
  dimension "d267" = 1.75
  dimension "d268" = 9.5
  constraints: 2 end point, 2 point on circle, 2 tangent, 1 centre point, 1 midpoint, 1 point on line, 1 vertical, 1 vertical alignment
  measures "d267" distance of L12.end A0.end
  measures "d268" vertical distance of point (-30.829, 17.325) A0.end
extrude "Vysunutí38" cut sketch "Náčrt27" against normal blind 12.2 contours A0 L13 | L12 L13 A0 | L13 A0
sketch "Náčrt28" plane through (33.6572, 33.5, 0) normal (0, 1, 0) x (1, 0, 0)
  line L0 (7.9222, -17.25) -> (7.9222, -13.25) projected
  line L1 (7.9222, -13.25) -> (-2.0778, -13.25) projected
  circle A0 centre (7.1722, -14) radius 0.75
  point P0 (-33.6572, 0)
  point P1 (7.1722, -13.25)
  point P2 (7.9222, -14)
  dimension "d271" = 1.5
  constraints: 2 tangent, 1 centre point
  measures "d271" diameter of A0
extrude "Vysunutí39" cut sketch "Náčrt28" against normal through all contours A0 L1 L0
sketch "Náčrt32" plane through (0, 0, 49.5) normal (0, 0, 1) x (1, 0, 0)
  arc A0 (29.0793, 0) -> (34.0793, 5) centre (29.0793, 5) ccw projected
  line L0 (34.0793, 5) -> (34.0793, 10) projected
  line L1 (0, 0) -> (29.0793, 0) projected
  circle A1 centre (29.0793, 5) radius 5
  line L2 (24.0793, 5) -> (24.0793, 0)
  line L3 (29.0793, 10) -> (34.0793, 10)
  circle A2 centre (29.0793, 5) radius 1.7
  line L4 (24.0793, 4.2) -> (19.6275, 4.2) projected
  line L5 (24.0793, 4.2) -> (24.1437, 4.2)
  point P0 (29.0793, 0)
  dimension "d281" = 3.4
  constraints: 6 end point, 4 point on circle, 2 centre point, 2 coincident, 2 perpendicular, 2 tangent, 1 horizontal, 1 point on line
  measures "d281" diameter of A2
extrude "Vysunutí43" cut sketch "Náčrt32" against normal blind 2 contours A1 A0 | L1 L2 L5 A1 | A1 L3 L0 | L5 L2 A1 | A2
extrude "Vysunutí44" cut sketch "Náčrt32" against normal up to next contours L1 L2 L5 A1 | A2
sketch "Náčrt33" plane through (0, 0, 44.9) normal (0, 0, -1) x (-1, 0, 0)
  arc A0 (-34.0793, 5) -> (-24.1437, 4.2) centre (-29.0793, 5) ccw projected
  arc A1 (-34.5793, 5) -> (-23.6378, 4.2) centre (-29.0793, 5) ccw
  line L0 (-24.1437, 4.2) -> (-19.6275, 4.2) projected
  line L1 (-24.0793, 0) -> (-24.0793, 4.2) projected
  line L2 (-24.0793, 0) -> (-29.0793, 0)
  arc A2 (-34.0793, 5) -> (-24.1437, 4.2) centre (-29.0793, 5) ccw projected
  arc A3 (-35.0793, 5) -> (-23.1329, 4.2) centre (-29.0793, 5) ccw
  line L3 (-23.5793, 4.2) -> (-20.5793, 4.2) projected
  point P0 (0, 0)
  point P1 (-24.0793, 2.7087)
  point P2 (-25.7627, 0)
  point P3 (-23.1329, 4.2)
  point P4 (-24.0793, 1.6834)
  dimension "d286" = 0.5
  dimension "d289" = 0.5
  constraints: 5 point on circle, 2 centre point, 2 end point, 2 horizontal alignment, 2 point on line, 1 horizontal
  measures "d286" radial gap between concentric circles of A0 A1
  measures "d289" radial gap between concentric circles of A1 A3
extrude "Vysunutí45" add sketch "Náčrt33" against normal up to surface (2.6 mm away) contours A0 L0 L1 A1 L2 | A1 L1 A3 L2 | L0 A1 L1 | A1 L0 A3 L1
extrude "Vysunutí46" add sketch "Náčrt33" against normal up to surface (3.6 mm away) contours L0 A1 L1 | A1 L0 A3 L1
sketch "Náčrt34" plane through (0, 0, 0) normal (0, -1, 0) x (1, 0, 0)
  line L0 (33.6572, 0) -> (27.3929, 0) projected
  line L1 (27.3929, 0) -> (-334.2817, 0) construction
  line L2 (-168.9876, 122.4745) -> (-72.395, 96.5926)
  line L3 (-72.395, 96.5926) -> (-98.2769, 0)
  line L4 (-98.2769, 0) -> (-194.8695, 25.8819)
  line L5 (-194.8695, 25.8819) -> (-168.9876, 122.4745)
  line L6 (30.8013, 33.0862) -> (34.2013, 38.9751) projected
  line L7 (32.5013, 36.0307) -> (-269.6449, 210.4749) construction
  circle A0 centre (40.7183, 0) radius 375
  point P0 (0, 0)
  point P1 (30.5041, 32.5713)
  point P2 (34.4986, 39.49)
  point P3 (-8.2817, 0)
  dimension "d292" = 100
  dimension "d293" = 15
  dimension "d296" = 49
  dimension "d297" = 750
  dimension "d298" = 30
  constraints: 12 end point, 3 perpendicular, 2 parallel, 2 point on circle, 2 point on line, 1 centre point, 1 coincident, 1 horizontal, 1 horizontal alignment, 1 midpoint
  measures "d292" distance of L4.end L2.start
  measures "d293" angle of L1 L4
  measures "d296" distance of point (40.718, 0) point (-8.282, 0)
  measures "d297" diameter of A0
  measures "d298" angle of L1 L7
sketch "Náčrt35" plane through (0, 0, 49.5) normal (0, 0, 1) x (1, 0, 0)
  line L0 (52.2183, 34) -> (52.2183, 35.6) construction
  line L1 (52.2183, 35.6) -> (89.7183, 35.6) construction
  line L2 (89.7183, 34) -> (52.2183, 34) construction
  line L3 (55.9683, 35.6) -> (55.9683, 34) construction
  line L4 (89.7183, 35.6) -> (89.7183, 34) construction
  circle A0 centre (74.2183, 15.5) radius 16.5 projected
  circle A1 centre (74.2183, 13.5) radius 16.5 construction
  circle A2 centre (74.2183, 11.5) radius 16.5 projected
  line L5 (57.7183, 15.5) -> (57.7183, 11.5) projected
  line L6 (49.1982, 33.5) -> (55.5315, 33.5) projected
  line L7 (39.8649, 10) -> (55.5315, 33.5) projected
  line L8 (55.5315, 33.5) -> (60.9683, 33.5)
  line L9 (60.9683, 33.5) -> (60.9683, 27.6)
  line L10 (60.9683, 27.6) -> (48.5961, 23.0969)
  line L11 (55.7748, 25.7097) -> (60.9683, 33.5)
  line L12 (50.9683, 33.5) -> (50.9683, 23.9603)
  point P0 (0, 0)
  point P1 (90.7183, 13.5)
  point P2 (50.9683, 26.6551)
  dimension "d299" = 5
  dimension "d300" = 8
  dimension "d301" = 70
  dimension "d304" = 5
  constraints: 10 end point, 4 point on line, 3 horizontal alignment, 1 horizontal, 1 parallel, 1 perpendicular, 1 vertical
  measures "d299" distance between parallel lines of L9 L3
  measures "d300" distance from line of L9.end L1
  measures "d301" angle of L10 L9
  measures "d304" distance between parallel lines of L12 L3
extrude "Vysunutí47" add sketch "Náčrt35" against normal blind 10.5 contours L6 L7 L12 | L8 L11 L10 L12 L7 | L12 L10 L7 | L9 L10 L11
extrude "Vysunutí49" cut sketch "Náčrt35" against normal blind 1.35 contours L9 L10 L11
sketch "Náčrt37" plane through (33.6572, 33.5, 0) normal (0, 1, 0) x (1, 0, 0)
  circle A0 centre (22.3111, -44.75) radius 1.65
  line L0 (17.3111, -39) -> (22.3111, -44.75) construction
  line L1 (22.3111, -44.75) -> (27.3111, -39) construction
  line L2 (18.5611, -39) -> (18.5611, -47.5)
  arc A1 (18.5611, -47.5) -> (19.5611, -48.5) centre (19.5611, -47.5) ccw
  line L3 (19.5611, -48.5) -> (27.3111, -48.5)
  line L4 (27.3111, -48.15) -> (27.3111, -39) projected
  line L5 (27.3111, -49.5) -> (27.3111, -48.15) projected
  line L6 (17.3111, -39) -> (27.3111, -39) projected
  line L7 (17.3111, -46.7924) -> (17.3111, -39) projected
  line L8 (15.541, -49.5) -> (27.3111, -49.5) projected
  arc A2 (17.6246, -47) -> (19.5611, -49.5) centre (19.5611, -47.5) ccw
  line L9 (17.3111, -47) -> (1.7643, -47) projected
  line L10 (17.6246, -47) -> (17.6246, -39)
  line L11 (27.3111, -39) -> (14.939, -39) projected
  point P0 (-33.6572, 0)
  dimension "d309" = 3.3
  dimension "d310" = 3.75
  dimension "d311" = 3.75
  dimension "d312" = 1
  dimension "d338" = 44.75
  constraints: 10 end point, 5 point on line, 4 point on circle, 3 centre point, 3 tangent, 2 vertical, 1 coincident, 1 equal length, 1 perpendicular
  measures "d309" diameter of A0
  measures "d310" distance from line of L3 L0.end
  measures "d311" distance from line of L2 L0.end
  measures "d312" radius of A1
  measures "d338" vertical distance of point (-33.657, 0) L0.end
extrude "Vysunutí50" add sketch "Náčrt37" along normal blind 2 contours L2 A1 L3 L5 L8 A2 L10 L6
ref_plane "Pracovní rovina16" through (50.9683, 26.6551, 39) normal (-0.8660254, 0, 0.5) x (0, -1, 0)
sketch "Náčrt39" plane through (50.9683, 26.6551, 39) normal (-0.8660254, 0, 0.5) x (0, -1, 0)
  line L0 (-6.8449, 0.625) -> (-6.8449, 5) projected
  line L1 (-0.9449, 5) -> (3.5582, -1.1861) projected
  line L2 (3.5582, -1.1861) -> (0, 0) projected
  line L3 (0, 0) -> (-6.8449, 0) projected
  line L4 (-6.8449, 0.1568) -> (-8.8449, 0.1568) projected
  line L5 (-6.6651, 6.9282) -> (0, 6.9282) projected
  line L6 (-6.8449, 6.7484) -> (-6.6651, 6.9282) projected
  line L7 (-6.8449, 6.7484) -> (-6.8449, 0) projected
  line L8 (0, 0) -> (-6.8449, 0) projected
  line L9 (0, 6.9282) -> (0, 0) projected
  line L10 (0, 6.9282) -> (3.5582, 5.7421) projected
  line L11 (0, 6.9282) -> (0, 0) projected
  line L12 (3.5582, -1.1861) -> (0, 0) projected
  line L13 (3.5582, 5.7421) -> (3.5582, -1.1861) projected
  line L14 (0, 0) -> (3.5582, 0)
  line L15 (-6.8449, 0) -> (-6.8449, 0.1568) projected
  line L16 (-8.8449, 0.625) -> (-8.8449, 0.1568) projected
  line L17 (-6.8449, 0.625) -> (-8.8449, 0.625) projected
  line L18 (-6.8449, 5) -> (-0.9449, 5) projected
  point P0 (26.6551, -59.2591)
  constraints: 2 end point, 1 perpendicular, 1 point on line
extrude "Vysunutí54" add sketch "Náčrt39" along normal up to next contours L0 L18 L1 L9 L3 L7 | L7 L6 L5 L9 L1 L18 | L9 L10 L13 L14 L1 | L1 L14 L9
sketch "Náčrt40" plane through (0, 0, 39) normal (0, 0, -1) x (-1, 0, 0)
  line L0 (-54.178, 25.1285) -> (-50.9683, 23.9603) projected
  line L1 (-53.8394, 23.0969) -> (-54.178, 25.1285) projected
  line L2 (-50.9683, 23.0969) -> (-53.8394, 23.0969) projected
  line L3 (-50.9683, 23.9603) -> (-50.9683, 23.0969) projected
  line L4 (-50.9683, 23.9603) -> (-48.5961, 23.0969) projected
  line L5 (-50.9683, 23.9603) -> (-48.5961, 23.0969) projected
  line L6 (-50.9683, 23.9603) -> (-50.9683, 23.0969) projected
  line L7 (-50.9683, 23.0969) -> (-48.5961, 23.0969) projected
  point P0 (0, 0)
extrude "Vysunutí55" cut sketch "Náčrt40" against normal through all
sketch "Náčrt41" plane through (48.5961, 23.0969, 39) normal (-0.8320503, 0.5547002, 0) x (0, 0, 1)
  point P0 (-39, -46.1741)
sketch "Náčrt42" plane through (33.6572, 35.5, 0) normal (0, 1, 0) x (1, 0, 0)
  line L0 (14.939, -40.3696) -> (17.3111, -39) projected
  line L1 (14.939, -39) -> (17.3111, -39) projected
  line L2 (14.939, -40.3696) -> (14.939, -39) projected
  point P0 (-33.6572, 0)
extrude "Vysunutí56" cut sketch "Náčrt42" against normal through all
sketch "Náčrt43" plane through (50.9683, 23.9603, 39) normal (-0.5, 0, -0.8660254) x (-0.8660254, 0, 0.5)
  line L0 (2.7391, -0.8634) -> (9.9024, -0.8634) projected
  line L1 (3.8962, 9.5397) -> (9.9024, -0.8634) projected
  line L2 (0, 0) -> (0, 9.5397) projected
  line L3 (2.7391, -0.8634) -> (0, 0) projected
  line L4 (0, 0) -> (0, 9.5397) projected
  line L5 (-1.0825, 9.5397) -> (-8.6603, 9.5397) projected
  line L6 (-8.6603, 3.6397) -> (0, 0) projected
  line L7 (2.7391, -0.8634) -> (11.4961, -3.6236)
  line L8 (9.9024, -0.8634) -> (17.4639, -13.9603) projected
  line L9 (-0.2715, 9.5397) -> (-0.2715, 11.5397) projected
  line L10 (0, 9.5397) -> (3.8962, 9.5397) projected
  line L11 (0, 9.5397) -> (-0.2715, 9.5397) projected
  line L12 (-1.0825, 11.5397) -> (-0.2715, 11.5397) projected
  line L13 (-1.0825, 9.5397) -> (-1.0825, 11.5397) projected
  line L14 (-8.6603, 9.5397) -> (-8.6603, 3.6397) projected
  point P0 (24.6398, -23.9603)
  constraints: 2 end point, 1 collinear, 1 point on line
extrude "Vysunutí57" add sketch "Náčrt43" against normal up to surface contours L0 L8 L7 surface through (44.5315, 21.75, 47) normal (0, 0, -1)
sketch "Náčrt44" plane through (0, 0, 49.5) normal (0, 0, 1) x (1, 0, 0)
  line L0 (48.5961, 23.0969) -> (47.7445, 21.8194) projected
  line L1 (47.7445, 21.8194) -> (52.4242, 23.0969) projected
  line L2 (52.4242, 23.0969) -> (48.5961, 23.0969) projected
  line L3 (60.9683, 29.1) -> (59.6479, 27.1194)
  line L4 (60.9683, 27.6) -> (50.9683, 23.9603) projected
  line L5 (55.7748, 25.7097) -> (60.9683, 33.5) projected
  line L6 (60.9683, 33.5) -> (60.9683, 27.6) projected
  point P0 (0, 0)
  dimension "d337" = 1.5
  constraints: 2 end point, 2 point on line, 1 parallel
  measures "d337" distance of L4.start L3.start
extrude "Vysunutí58" cut sketch "Náčrt44" against normal through all contours L2 L1 L0 | L6 L4 L3
extrude "Vysunutí51" cut sketch "Náčrt37" against normal through all contours A0
ref_plane "Pracovní rovina14" through (33.6572, 30.5, 0) normal (0, 1, 0) x (1, 0, 0)
sketch "Náčrt38" plane through (33.6572, 30.5, 0) normal (0, 1, 0) x (1, 0, 0)
  circle A0 centre (22.3111, -44.75) radius 1.65 projected
  line L0 (23.8989, -42) -> (25.4866, -44.75)
  line L1 (25.4866, -44.75) -> (23.8989, -47.5)
  line L2 (23.8989, -47.5) -> (20.7234, -47.5)
  line L3 (20.7234, -47.5) -> (19.1357, -44.75)
  line L4 (19.1357, -44.75) -> (20.7234, -42)
  line L5 (20.7234, -42) -> (23.8989, -42)
  point P0 (-33.6572, 0)
  dimension "d318" = 5.5
  constraints: 12 end point, 1 coincident, 1 horizontal, 13 other
  measures "d318" distance between parallel lines of L2 L5
extrude "Vysunutí52" cut sketch "Náčrt38" against normal through all contours A0 | L0 L1 L2 L3 L4 L5
chamfer "Zkosení1" distance 0.75 angle 45 1 edges at (54.3183, 30.5, 44.75)
extrude "Vysunutí53" add sketch "Náčrt37" along normal blind 0.5 contours L6 L4 L5 L3 A1 L2
mirror "Zrcadlit1" about plane through (28.5277, 7.75, 0) normal (0, 0, -1)
